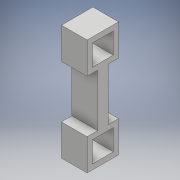
# Autodesk Inventor part: extenstion
Saved by Autodesk Inventor 2018 (Build 220112000, 112)
## iProperties
Created: 2018-01-21
Part Number: extenstion
Material: Generic
Document SubType Name: Modeling
Designer: omara
Density: 1 g/cm^3
Appearance: Default
Author: omara
Autodesk Inventor part; units mm, degrees
ref_plane "YZ Plane" through (0, 0, 0) normal (1, 0, 0) x (0, 1, 0)
ref_plane "XZ Plane" through (0, 0, 0) normal (0, 1, 0) x (-1, 0, 0)
ref_plane "XY Plane" through (0, 0, 0) normal (0, 0, 1) x (1, 0, 0)
sketch "Sketch1" plane through (0, 0, 0) normal (1, 0, 0) x (0, 1, 0)
  point P0 (0, 0)
sketch "Sketch2" plane through (0, 0, 0) normal (1, 0, 0) x (0, 1, 0)
  line L0 (0, 0) -> (20, 0)
  line L1 (20, 0) -> (20, -100)
  line L2 (20, -100) -> (0, -100)
  line L3 (0, -100) -> (0, 0)
  line L4 (40, 60) -> (-20, 60)
  line L5 (-20, 60) -> (-20, 0)
  line L6 (-20, 0) -> (40, 0)
  line L7 (40, 0) -> (40, 60)
  line L8 (40, -100) -> (-20, -100)
  line L9 (-20, -100) -> (-20, -160)
  line L10 (-20, -160) -> (40, -160)
  line L11 (40, -160) -> (40, -100)
  line L12 (30, 50) -> (-10, 50)
  line L13 (-10, 50) -> (-10, 10)
  line L14 (-10, 10) -> (30, 10)
  line L15 (30, 10) -> (30, 50)
  line L16 (30, -110) -> (-10, -110)
  line L17 (-10, -110) -> (-10, -150)
  line L18 (-10, -150) -> (30, -150)
  line L19 (30, -150) -> (30, -110)
  dimension "d0" = 100
  dimension "d1" = 20
  dimension "d2" = 60
  dimension "d3" = 60
  dimension "d4" = 0
  dimension "d5" = 20
  dimension "d6" = 60
  dimension "d7" = 40
  dimension "d8" = 40
  dimension "d9" = 10
  dimension "d10" = 10
  dimension "d11" = 40
  dimension "d12" = 40
  dimension "d13" = 10
  dimension "d14" = 10
  constraints: 40 end point, 10 parallel, 5 horizontal, 5 perpendicular, 1 point on line
  measures "d0" distance of L0.end L1.end
  measures "d1" distance of L1.end L2.end
  measures "d2" distance of L6.end L5.end
  measures "d3" distance of L4.end L5.end
  measures "d4" distance between parallel lines of L0 L6
  measures "d5" distance between parallel lines of L7 L1
  measures "d6" distance of L8.end L9.end
  measures "d7" distance of L14.end L13.end
  measures "d8" distance of L12.end L13.end
  measures "d9" distance between parallel lines of L4 L12
  measures "d10" distance between parallel lines of L7 L15
  measures "d11" distance of L16.end L17.end
  measures "d12" distance of L16.start L16.end
  measures "d13" distance between parallel lines of L10 L18
  measures "d14" distance between parallel lines of L9 L17
extrude "Extrusion1" add sketch "Sketch2" along normal blind 49
body "Solid1"
